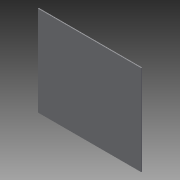
# Autodesk Inventor part: Aluminum Mount Plate
Saved by Autodesk Inventor 2015 (Build 190159000, 159)
## iProperties
Created: 2015-01-11
Part Number: Aluminum Mount Plate
Material: Generic
Document SubType Name: Modeling
Designer: jhirshland1
Density: 1 g/cm^3
Appearance: Default
Author: jhirshland1
Autodesk Inventor part; units mm, degrees
ref_plane "YZ Plane" through (0, 0, 0) normal (1, 0, 0) x (0, 1, 0)
ref_plane "XZ Plane" through (0, 0, 0) normal (0, 1, 0) x (-1, 0, 0)
ref_plane "XY Plane" through (0, 0, 0) normal (0, 0, 1) x (1, 0, 0)
sketch "Sketch1" plane through (0, 0, 0) normal (0, 0, 1) x (1, 0, 0)
  line L0 (-593.8051, 5.0592) -> (104.6949, 5.0592)
  line L1 (104.6949, 5.0592) -> (104.6949, -604.5408)
  line L2 (104.6949, -604.5408) -> (-593.8051, -604.5408)
  line L3 (-593.8051, -604.5408) -> (-593.8051, 5.0592)
  point P0 (0, 0)
  dimension "d0" = 698.5
  dimension "d1" = 609.6
  constraints: 8 end point, 2 parallel, 1 horizontal, 1 perpendicular
  measures "d0" distance of L1.end L2.end
  measures "d1" distance of L0.end L1.end
extrude "Extrusion1" add sketch "Sketch1" against normal blind 6.35
body "Solid1"
